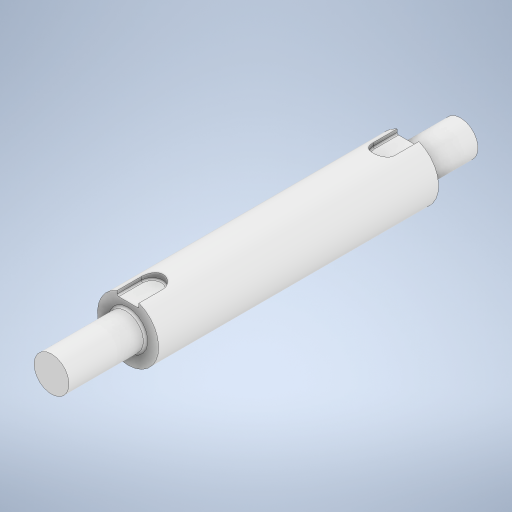
# Autodesk Inventor part: eje1
Saved by Autodesk Inventor 2024.3 (Build 283343000, 343)
## iProperties
Created: 2024-05-18
Part Number: eje1
Material: PBT Plastic
Document SubType Name: Modeling
Designer: USUARIO
Density: 1.31 g/cm^3
Appearance: Smooth - White
Mass: 18.2972 g
Surface Area: 42.7857 cm^2
Volume: 13.9673 cm^3
Author: USUARIO
Autodesk Inventor part; units mm, degrees
ref_plane "YZ Plane" through (0, 0, 0) normal (1, 0, 0) x (0, 1, 0)
sketch "Sketch1" plane through (0, 0, 0) normal (1, 0, 0) x (0, 1, 0)
  line L0 (0, 0) -> (7, 0)
  line L1 (7, 0) -> (7, -64)
  line L2 (7, -64) -> (0, -64)
  line L3 (0, 0) -> (0, -64)
  line L4 (0, 18.3308) -> (0, -79.8767)
  line L5 (0, -64) -> (4, -64)
  line L6 (4, -64) -> (4, -76)
  line L7 (4, -76) -> (4, -76)
  line L8 (0, -76) -> (0, -74)
  line L9 (0, -76) -> (4, -76)
  line L10 (0, -74) -> (0, -76)
  line L11 (4, -76) -> (0, -76)
  line L12 (0, -74) -> (0, -64)
  line L13 (0, 0) -> (4, 0)
  line L14 (4, 0) -> (4, 17.5)
  line L15 (4, 17.5) -> (0, 17.5)
  line L16 (0, 17.5) -> (0, 0)
  point P0 (0, -82)
  point P1 (0, -64)
  point P2 (0, 17.5)
  point P3 (4, 0)
  point P4 (0, -76)
  dimension "d0" = 7
  dimension "d1" = 64
  dimension "d7" = 12
  dimension "d11" = 4
  dimension "d35" = 4
  dimension "d36" = 17.5
  constraints: 34 end point, 6 parallel, 4 horizontal, 3 perpendicular, 2 point on line, 2 vertical
  measures "d0" distance of L0.start L0.end
  measures "d1" distance of L0.end L1.end
  measures "d7" distance of L5.end L6.end
  measures "d11" distance of L6.end L8.start
  measures "d35" distance of L15.end L14.end
  measures "d36" distance of L14.end L13.end
ref_plane "Work Plane1" through (0, 0, 14.5) normal (0, 0, 1) x (1, 0, 0)
revolve "Revolution2" add sketch "Sketch1" angle 360 about axis through (0, 0, 18.3308) along (0, 0, -1)
sketch "Sketch4" plane through (0, 0, 0) normal (0, 0, 1) x (1, 0, 0)
  line L0 (0, 7) -> (2.5, 7)
  line L1 (2.5, 7) -> (-2.5, 7)
  line L2 (-2.5, 7) -> (-2.5, 5.5)
  line L3 (-2.5, 5.5) -> (2.5, 5.5)
  line L4 (2.5, 5.5) -> (2.5, 7)
  circle A0 centre (0, 0) radius 7 projected
  point P0 (0, 0)
  point P1 (0, 7)
  dimension "d37" = 2.5
  dimension "d38" = 5
  dimension "d39" = 1.5
  constraints: 10 end point, 2 horizontal, 2 midpoint, 2 parallel, 1 perpendicular, 1 vertical alignment, 1 other
  measures "d37" distance of L0.start L0.end
  measures "d38" distance of L3.end L2.end
  measures "d39" distance of L2.end L1.end
extrude "Extrusion5" cut sketch "Sketch4" against normal blind 5.5 contours A0 L2 L1 | L0 L4 A0 | A0 L4 L3 L2 picked at (0, 6)
sketch "Sketch5" plane through (0, 0, -64) normal (0, 0, -1) x (-1, 0, 0)
  line L0 (0, 7) -> (2.5, 7)
  line L1 (2.5, 7) -> (-2.5, 7)
  line L2 (-2.5, 7) -> (-2.5, 5.5)
  line L3 (-2.5, 5.5) -> (2.5, 5.5)
  line L4 (2.5, 5.5) -> (2.5, 7)
  circle A0 centre (0, 0) radius 7 projected
  point P0 (0, 0)
  point P1 (0, 7)
  dimension "d42" = 2.5
  dimension "d43" = 5
  dimension "d44" = 1.5
  constraints: 10 end point, 2 horizontal, 2 midpoint, 2 parallel, 1 perpendicular, 1 vertical alignment, 1 other
  measures "d42" distance of L0.start L0.end
  measures "d43" distance of L3.end L2.end
  measures "d44" distance of L2.end L1.end
extrude "Extrusion6" cut sketch "Sketch5" against normal blind 5.5 contours A0 L2 L1 | L0 L4 A0 | A0 L4 L3 L2 picked at (0, 6)
ref_plane "Work Plane2" through (0, 7, -32) normal (0, 1, 0) x (1, 0, 0)
sketch "Sketch6" plane through (0, 7, -32) normal (0, 1, 0) x (1, 0, 0)
  line L0 (2.5, -26.5) -> (-2.5, -26.5) projected
  circle A0 centre (0, -26.5) radius 2.5
  line L1 (-2.5, 26.5) -> (2.5, 26.5) projected
  circle A1 centre (0, 26.5) radius 2.5
  point P0 (0, -32)
  constraints: 2 horizontal alignment, 2 midpoint, 4 other
extrude "Extrusion7" cut sketch "Sketch6" against normal blind 1.5
fillet "Fillet4" radius 0.35 6 edges at (0, 5.5, -8) (2.5, 5.5, -2.75) (-2.5, 5.5, -2.75) (-2.5, 5.5, -61.25) (2.5, 5.5, -61.25) (0, 5.5, -56)
fillet "Fillet5" radius 0.5 2 edges at (0, -4, 0) (0, -4, -64)
body "Solid1"
